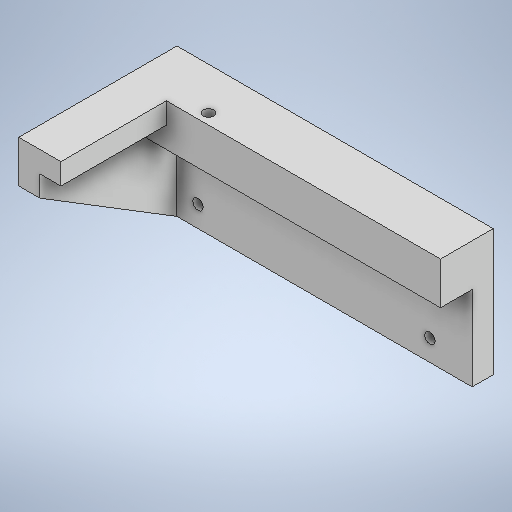
# Autodesk Inventor part: ModuleConnector
Saved by Autodesk Inventor 2025.3 (Build 293356000, 356)
## iProperties
Created: 2025-04-27
Part Number: ModuleConnector
Material: 일반
Document SubType Name: Modeling
Designer: SEON
Density: 1 g/cm^3
Appearance: 기본값
Author: SEON
Autodesk Inventor part; units mm, degrees
ref_plane "YZ Plane" through (0, 0, 0) normal (1, 0, 0) x (0, 1, 0)
sketch "스케치1" plane through (0, 0, 0) normal (0, 0, 1) x (1, 0, 0)
  line L0 (0, 10) -> (0, 0)
  line L1 (-10, 10) -> (-10, 20)
  line L2 (-10, 20) -> (290, 20)
  line L3 (290, 20) -> (290, 10)
  line L4 (0, 0) -> (280, 0)
  line L5 (290, 10) -> (290, -40)
  line L6 (-10, 10) -> (-10, -40)
  line L7 (-10, -40) -> (290, -40)
  line L8 (0, 10) -> (10, 10)
  line L9 (10, 10) -> (10, 20)
  line L10 (140, 20) -> (140, 10)
  line L11 (0, 0) -> (-10, 0)
  line L12 (280, 10) -> (280, 0)
  line L13 (280, 10) -> (270, 10)
  line L14 (270, 10) -> (270, 20)
  line L15 (280, 0) -> (290, 0)
  point P0 (140, 0)
  dimension "d2" = 10
  dimension "d5" = 10
  dimension "d6" = 300
  dimension "d9" = 60
  dimension "d12" = 10
  dimension "d13" = 10
  constraints: 32 end point, 5 perpendicular, 4 symmetric about line, 3 vertical, 2 horizontal, 2 midpoint, 2 point on line, 1 coincident, 1 vertical alignment
  measures "d2" distance of L0.start L0.end
  measures "d5" distance between parallel lines of L0 L1
  measures "d6" distance of L1.end L2.end
  measures "d9" distance between parallel lines of L2 L7
  measures "d12" distance of L0.start L8.end
  measures "d13" distance of L8.end L9.end
extrude "돌출1" add sketch "스케치1" along normal blind 25 contours L8 L9 L2 L14 L13 L12 L4 L0 | L0 L11 L6 L1 L2 L9 L8 | L12 L13 L14 L2 L3 L5 L15
extrude "돌출2" add sketch "스케치1" along normal blind 10 contours L8 L9 L2 L14 L13 L12 L4 L0 | L4 L15 L5 L7 L6 L11
extrude "돌출3" add sketch "스케치1" along normal blind 75 contours L0 L11 L6 L1 L2 L9 L8 | L12 L13 L14 L2 L3 L5 L15
sketch "스케치2" plane through (-10, -40, 0) normal (-1, 0, 0) x (0, 0, 1)
  line L0 (0, 60) -> (0, 0) projected
  line L1 (0, 0) -> (10, 0) projected
  line L2 (10, 40) -> (10, 0) projected
  line L3 (10, 40) -> (75, 40) projected
  line L4 (75, 60) -> (75, 40) projected
  line L5 (0, 60) -> (75, 60) projected
  line L6 (75, 40) -> (10, 0)
  point P0 (0, 40)
  constraints: 2 end point
extrude "돌출4" add sketch "스케치2" against normal up to surface (10 mm away) contours L2 L3 L6
ref_plane "작업 평면1" through (140, -40, 0) normal (1, 0, 0) x (0, 0, -1)
mirror "미러1" about plane through (140, -40, 0) normal (1, 0, 0) of "돌출4"
sketch "스케치3" plane through (0, 0, 10) normal (0, 0, 1) x (1, 0, 0)
  circle A0 centre (10, -10) radius 2.5
  circle A1 centre (120, -10) radius 2.5
  line L0 (270, 20) -> (10, 20) projected
  line L1 (290, -40) -> (290, 0) projected
  line L2 (-10, -40) -> (-10, 0) projected
  circle A2 centre (10, -30) radius 2.5
  circle A3 centre (120, -30) radius 2.5
  line L3 (140, 20) -> (140, -20)
  point P0 (0, 0)
  dimension "d18" = 30
  dimension "d19" = 5
  dimension "d21" = 20
  dimension "d24" = 5
  dimension "d25" = 20
  dimension "d38" = 20
  constraints: 4 centre point, 2 end point, 2 equal radius, 2 horizontal alignment, 2 vertical alignment, 1 midpoint, 1 vertical
  measures "d18" distance from line of L0 A1.centre
  measures "d19" diameter of A1
  measures "d21" distance from line of L2 A0.centre
  measures "d24" diameter of A3
  measures "d25" distance of A0.centre A2.centre
  measures "d38" distance from line of A3.centre L3
extrude "돌출5" cut sketch "스케치3" against normal through all
sketch "스케치4" plane through (-10, 20, 0) normal (0, 1, 0) x (1, 0, 0)
  line L0 (280, -25) -> (280, -75) projected
  line L1 (20, -25) -> (20, -75) projected
  line L2 (280, -25) -> (20, -25) projected
  point P0 (10, 0)
  point P1 (35, -20)
  point P2 (265, -20)
  dimension "d26" = 15
  dimension "d27" = 15
  dimension "d28" = 5
  constraints: 1 horizontal alignment
  measures "d26" distance from line of L0 point (265, -20)
  measures "d27" distance from line of L1 point (35, -20)
  measures "d28" distance from line of L2 point (265, -20)
hole "구멍1" at (25, 20, 20) at (255, 20, 20) direction (0, -1, 0) diameter 3 end through all counterbore diameter 5 counterbore depth 5
ref_plane "작업 평면2" through (140, -40, 0) normal (1, 0, 0) x (0, 0, -1)
sketch "스케치5" plane through (140, -40, 0) normal (1, 0, 0) x (0, 0, -1)
  line L0 (0, 0) -> (-10, 0) projected
  line L1 (0, 0) -> (0, 60) projected
  line L2 (0, 60) -> (-75, 60) projected
  line L3 (-75, 40) -> (-75, 60) projected
  line L4 (-10, 0) -> (-75, 40) projected
  point P0 (0, 40)
extrude "돌출6" cut sketch "스케치5" along normal through all
